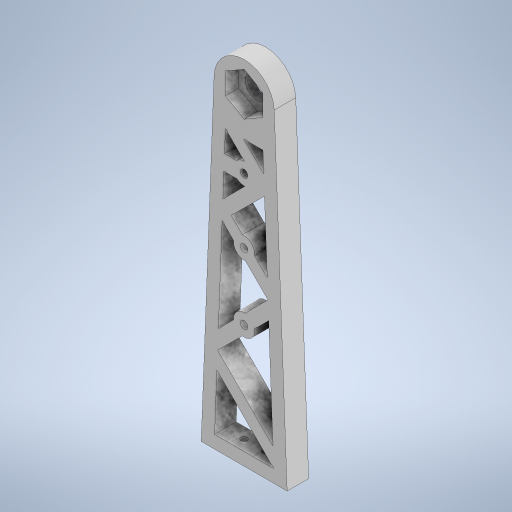
# Autodesk Inventor part: 전체 형상
Saved by Autodesk Inventor 2023 (Build 270158000, 158)
## iProperties
Created: 2022-11-11
Part Number: 전체 형상
Material: 일반
Document SubType Name: Modeling
Designer: hyunsu
Density: 1 g/cm^3
Appearance: 기본값
Author: hyunsu
Autodesk Inventor part; units mm, degrees
ref_plane "YZ Plane" through (0, 0, 0) normal (1, 0, 0) x (0, 1, 0)
ref_plane "XZ Plane" through (0, 0, 0) normal (0, 1, 0) x (-1, 0, 0)
ref_plane "XY Plane" through (0, 0, 0) normal (0, 0, 1) x (1, 0, 0)
sketch "스케치1" plane through (0, 0, 0) normal (0, 0, 1) x (1, 0, 0)
  line L0 (-5, -33) -> (5, -33)
  line L1 (5, -33) -> (5, 33)
  line L2 (5, 33) -> (-5, 33)
  line L3 (-5, 33) -> (-5, -33)
  line L4 (-5, -33) -> (5, 33) construction
  line L5 (5, -33) -> (-5, 33) construction
  line L6 (-5, 33) -> (-35, 33)
  line L7 (-35, 33) -> (-35, 23)
  line L8 (-35, 23) -> (-5, 23)
  line L9 (-5, 23) -> (-5, 33)
  line L10 (0, 0) -> (-11.0402, 0)
  line L11 (-5, -33) -> (-35, -33)
  line L12 (-35, -33) -> (-35, -23)
  line L13 (-35, -23) -> (-5, -23)
  point P0 (-5, 23)
  point P1 (-5, -23)
  dimension "d0" = 66
  dimension "d1" = 10
  dimension "d2" = 10
  dimension "d3" = 30
  constraints: 28 end point, 4 parallel, 3 horizontal, 3 symmetric about line, 2 midpoint, 2 perpendicular
  measures "d0" distance of L0.end L1.end
  measures "d1" distance of L1.end L2.end
  measures "d2" distance of L6.end L7.end
  measures "d3" distance of L2.end L6.end
extrude "돌출1" add sketch "스케치1" along normal mid plane 50
sketch "스케치2" plane through (0, 0, 25) normal (0, 0, 1) x (1, 0, 0)
  circle A0 centre (-15, 183) radius 14
  line L0 (-35, 33) -> (-35, 23) projected
  line L1 (-35, 33) -> (-28.9889, 183.5585)
  line L2 (5, 33) -> (-35, 33) projected
  line L3 (-15, 33) -> (-15, 183) construction
  line L4 (5, 33) -> (-1.0111, 183.5585)
  point P0 (0, 0)
  dimension "d6" = 28
  dimension "d7" = 150
  constraints: 6 end point, 1 coincident, 1 midpoint, 1 symmetric about line, 1 vertical, 4 other
  measures "d7" distance of L3.start L3.end
extrude "돌출2" add sketch "스케치2" against normal blind 10
ref_plane "작업 평면1" through (-15, 23, -25) normal (-1, 0, 0) x (0, 0, 1)
sketch "스케치3" plane through (-15, 23, -25) normal (-1, 0, 0) x (0, 0, 1)
  line L0 (40, 160.5585) -> (40, 10) projected
  line L1 (0, 10) -> (40, 10) projected
  line L2 (40, 144.5585) -> (0, 10)
  line L3 (45.7513, 142.8488) -> (8.0431, 16)
  line L4 (8.0431, 16) -> (34, 16)
  line L5 (34, 16) -> (34, 160.5585)
  line L6 (34, 16) -> (20, 56.2226)
  line L7 (34, 34.2526) -> (22.9265, 66.0672)
  point P0 (25, -23)
  point P1 (34, 103.318)
  point P2 (34, 124.3747)
  point P3 (40, 123.5018)
  dimension "d10" = 16
  dimension "d11" = 6
  dimension "d12" = 6
  constraints: 12 end point, 4 point on line, 1 parallel, 2 other
  measures "d10" distance of L0.start L2.start
  measures "d11" distance between parallel lines of L2 L3
  measures "d12" distance between parallel lines of L6 L7
extrude "돌출3" add sketch "스케치3" along normal mid plane 10 contours L0 L3 L5 L2 | L0 L1 L2 L5 L3 | L7 L5 L6 L3
sketch "스케치4" plane through (0, 0, 25) normal (0, 0, 1) x (1, 0, 0)
  line L0 (-35, 33) -> (-28.9889, 183.5585) projected
  line L1 (5, 33) -> (-1.0111, 183.5585) projected
  line L2 (-35, 33) -> (5, 33)
  arc A0 (-1.0111, 183.5585) -> (-28.9889, 183.5585) centre (-15, 183) ccw projected
  line L3 (-7.0064, 183.3192) -> (-1.2443, 39)
  line L4 (-1.2443, 39) -> (-28.7557, 39)
  line L5 (-28.7557, 39) -> (-22.9936, 183.3192)
  arc A1 (-7.0064, 183.3192) -> (-22.9936, 183.3192) centre (-15, 183) ccw
  line L6 (-1.2443, 39) -> (-27.6994, 65.4551)
  line L7 (-1.5972, 47.8382) -> (-27.3737, 73.6146)
  line L8 (-27.3737, 73.6146) -> (-3.5765, 97.4118)
  line L9 (-3.9022, 105.5713) -> (-27.0208, 82.4528)
  line L10 (-3.9022, 105.5713) -> (-25.2456, 126.9147)
  line L11 (-25.2456, 126.9147) -> (-5.5411, 146.6192)
  line L12 (-5.5411, 146.6192) -> (-23.7326, 164.8107)
  line L13 (-23.7326, 164.8107) -> (-6.2674, 164.8107)
  line L14 (-21.003, 131.1573) -> (-4.2551, 114.4095)
  line L15 (-15.2473, 164.8107) -> (-5.894, 155.4574)
  line L16 (-24.8927, 135.7528) -> (-9.7837, 150.8618)
  point P0 (0, 0)
  point P1 (-5.2153, 138.4597)
  dimension "d15" = 6
  dimension "d16" = 45
  dimension "d17" = 6
  dimension "d18" = 90
  dimension "d19" = 6
  dimension "d23" = 6
  constraints: 28 end point, 9 point on line, 3 parallel, 3 perpendicular, 2 horizontal, 2 point on circle, 1 centre point, 14 other
  measures "d16" angle of L4 L6
  measures "d17" distance between parallel lines of L6 L7
  measures "d18" angle of L7 L8
  measures "d19" distance between parallel lines of L8 L9
  measures "d23" distance between parallel lines of L16 L11
extrude "돌출4" cut sketch "스케치4" against normal blind 10 contours L3 L15 L13 | L12 L16 L5 | L3 L14 L11 | L10 L9 L5 | L3 L7 L8 | L6 L4 L5
sketch "스케치5" plane through (5, -33, -25) normal (1, 0, 0) x (0, 0, -1)
  line L0 (0, 66) -> (0, 0) projected
  line L1 (0, 66) -> (-101.2594, 66)
  line L2 (-101.2594, 66) -> (-101.2594, -7.0647)
  line L3 (-101.2594, -7.0647) -> (0, -7.0647)
  line L4 (0, -7.0647) -> (0, 66)
  point P0 (-25, 33)
  constraints: 8 end point, 2 parallel, 1 horizontal, 1 perpendicular
extrude "돌출5" cut sketch "스케치5" against normal blind 149
sketch "스케치6" plane through (-10, 23, -25) normal (1, 0, 0) x (0, 0, -1)
  line L0 (-40, 10) -> (-40, 16) projected
  line L1 (-40, 10) -> (44.1562, 10)
  line L2 (44.1562, 10) -> (44.1562, 152.029)
  line L3 (44.1562, 152.029) -> (-40, 152.029)
  line L4 (-40, 152.029) -> (-40, 10)
  point P0 (-25, -23)
  constraints: 8 end point, 2 parallel, 1 horizontal, 1 perpendicular
extrude "돌출6" cut sketch "스케치6" against normal blind 149
ref_plane "작업 평면2" through (-15, 533.9312, 25) normal (1, 0, 0) x (0, 0, -1)
sketch "스케치7" plane through (-15, 533.9312, 25) normal (1, 0, 0) x (0, 0, -1)
  line L0 (10, -350.3727) -> (10, -336.9312) projected
  circle A0 centre (10, -339.3727) radius 1
  line L1 (0, -350.3727) -> (10, -350.3727) projected
  point P0 (25, -533.9312)
  point P1 (10, -338.3727)
  point P2 (10, -340.3727)
  dimension "d28" = 2
  dimension "d29" = 11
  constraints: 1 centre point, 1 point on line
  measures "d28" diameter of A0
  measures "d29" distance from line of A0.centre L1
revolve "회전1" add sketch "스케치7" angle 360 about axis through (-15, 183.5585, 15) along (0, 1, 0) picked at (10.3333, -339.3727) contours L0 A0
sketch "스케치8" plane through (0, 0, 15) normal (0, 0, -1) x (-1, 0, 0)
  arc A0 (28.9889, 183.5585) -> (1.0111, 183.5585) centre (15, 183) ccw projected
  circle A1 centre (15, 183) radius 5.5
  point P0 (0, 0)
  dimension "d31" = 11
  constraints: 1 centre point, 1 coincident
  measures "d31" diameter of A1
extrude "돌출7" cut sketch "스케치8" against normal blind 149
sketch "스케치9" plane through (0, 0, 25) normal (0, 0, 1) x (1, 0, 0)
  circle A0 centre (-15, 183) radius 5.5 projected
  line L0 (-15, 193.0459) -> (-6.3, 188.0229)
  line L1 (-6.3, 188.0229) -> (-6.3, 177.9771)
  line L2 (-6.3, 177.9771) -> (-15, 172.9541)
  line L3 (-15, 172.9541) -> (-23.7, 177.9771)
  line L4 (-23.7, 177.9771) -> (-23.7, 188.0229)
  line L5 (-23.7, 188.0229) -> (-15, 193.0459)
  point P0 (0, 0)
  dimension "d34" = 17.4
  constraints: 12 end point, 1 coincident, 13 other
  measures "d34" distance between parallel lines of L1 L4
extrude "돌출8" cut sketch "스케치9" against normal blind 6
pattern_circular "원형 패턴1" count 20 over 360 about axis through (-15, 183, 15) along (0, 0, 1) of "회전1"
sketch "스케치12" plane through (-35, 33, 15) normal (0, -1, 0) x (1, 0, 0)
  circle A0 centre (35, 5) radius 1.5
  line L0 (40, 0) -> (40, 10) projected
  line L1 (0, 10) -> (40, 10) projected
  circle A1 centre (25, 5) radius 1.5
  circle A2 centre (15, 5) radius 1.5
  point P0 (35, -15)
  dimension "d54" = 3
  dimension "d55" = 5
  dimension "d58" = 10
  constraints: 3 centre point, 1 horizontal, 4 other
  measures "d54" diameter of A0
  measures "d55" distance from line of L0 A0.centre
  measures "d58" distance of A0.centre A1.centre
extrude "돌출11" cut sketch "스케치12" against normal blind 10
sketch "스케치13" plane through (0, 0, 15) normal (0, 0, -1) x (-1, 0, 0)
  line L0 (-7.0292, 147.2176) -> (26.5967, 147.2176)
  line L1 (26.5967, 147.2176) -> (26.5967, 154.5061)
  line L2 (26.5967, 154.5061) -> (-7.0292, 154.5061)
  line L3 (-7.0292, 154.5061) -> (-7.0292, 147.2176)
  line L4 (9.7837, 150.8618) -> (24.8927, 135.7528) projected
  line L5 (-7.0292, 147.2176) -> (26.5967, 154.5061) construction
  line L6 (26.5967, 147.2176) -> (-7.0292, 154.5061) construction
  line L7 (23.7326, 164.8107) -> (9.7837, 150.8618) projected
  line L8 (23.7326, 164.8107) -> (24.8927, 135.7528) projected
  point P0 (0, 0)
  point P1 (24.435, 147.2176)
  point P2 (24.144, 154.5061)
  point P3 (13.428, 154.5061)
  point P4 (13.428, 147.2176)
  constraints: 12 end point, 2 midpoint, 2 parallel, 1 horizontal, 1 perpendicular
extrude "돌출12" add sketch "스케치13" against normal blind 10 contours L4 L7 L2 L8 L0
sketch "스케치14" plane through (0, 0, 15) normal (0, 0, -1) x (-1, 0, 0)
  line L0 (35, 33) -> (-5, 33) projected
  circle A0 centre (15, 183) radius 5.5 projected
  line L1 (15, 33) -> (15, 183) construction
  circle A1 centre (15, 151) radius 1.75
  circle A2 centre (15, 121) radius 1.75
  circle A3 centre (15, 90) radius 1.75
  circle A4 centre (15, 151) radius 5
  circle A5 centre (15, 121) radius 5
  circle A6 centre (15, 90) radius 5
  point P0 (0, 0)
  dimension "d67" = 3.5
  dimension "d68" = 3.5
  dimension "d69" = 3.5
  dimension "d70" = 30
  dimension "d71" = 31
  dimension "d72" = 57
  dimension "d75" = 10
  dimension "d76" = 10
  dimension "d77" = 10
  constraints: 6 centre point, 3 coincident, 3 point on line, 2 end point, 1 midpoint
  measures "d67" diameter of A1
  measures "d68" diameter of A2
  measures "d69" diameter of A3
  measures "d70" distance of A2.centre A1.centre
  measures "d71" distance of A3.centre A2.centre
  measures "d72" distance from line of L0 A3.centre
  measures "d75" diameter of A4
  measures "d76" diameter of A5
  measures "d77" diameter of A6
extrude "돌출13" cut sketch "스케치14" against normal blind 10 contours A1 | A2 | A3
extrude "돌출14" add sketch "스케치14" against normal blind 10 contours A4 | A5 | A6
sketch "스케치15" plane through (0, 0, 15) normal (0, 0, -1) x (-1, 0, 0)
  circle A0 centre (15, 90) radius 1.75 projected
  circle A1 centre (15, 90) radius 3
  circle A2 centre (15, 121) radius 1.75 projected
  circle A3 centre (15, 121) radius 3
  circle A4 centre (15, 151) radius 1.75 projected
  circle A5 centre (15, 151) radius 3
  point P0 (0, 0)
  dimension "d80" = 6
  dimension "d81" = 6
  dimension "d82" = 6
  constraints: 3 centre point, 3 coincident
  measures "d80" diameter of A1
  measures "d81" diameter of A3
  measures "d82" diameter of A5
extrude "돌출15" cut sketch "스케치15" against normal blind 2.5 contours A0 | A1 | A2 | A3 | A4 | A5
